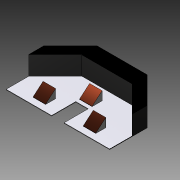
# Autodesk Inventor part: Charging Dock
Saved by Autodesk Inventor 2018 (Build 220112000, 112)
## iProperties
Created: 2017-03-09
Part Number: Charging Dock
Material: ABS Plastic
Document SubType Name: Modeling
Designer: Eightfold_Infotech
Density: 1.06 g/cm^3
Appearance: Smooth - White
Author: Eightfold_Infotech
Autodesk Inventor part; units mm, degrees
ref_plane "YZ Plane" through (0, 0, 0) normal (1, 0, 0) x (0, 1, 0)
ref_plane "XZ Plane" through (0, 0, 0) normal (0, 1, 0) x (-1, 0, 0)
ref_plane "XY Plane" through (0, 0, 0) normal (0, 0, 1) x (1, 0, 0)
sketch "Sketch1" plane through (0, 0, 0) normal (0, 1, 0) x (-1, 0, 0)
  line L0 (-50, -60.443) -> (50, -60.443)
  line L1 (50, -60.443) -> (50, 19.557)
  line L2 (50, 19.557) -> (-50, 19.557)
  line L3 (-50, 19.557) -> (-50, -60.443)
  line L4 (-50, -60.443) -> (50, 19.557) construction
  line L5 (50, -60.443) -> (-50, 19.557) construction
  line L6 (-250, 190) -> (-150, 190)
  line L7 (-150, 190) -> (-150, 110)
  line L8 (-150, 110) -> (-250, 110)
  line L9 (-250, 110) -> (-250, 190)
  line L10 (-250, 190) -> (-150, 110) construction
  line L11 (-150, 190) -> (-250, 110) construction
  line L12 (0, 214.4175) -> (0, -235.835)
  line L13 (250, 190) -> (150, 190)
  line L14 (150, 190) -> (150, 110)
  line L15 (150, 110) -> (250, 110)
  line L16 (250, 110) -> (250, 190)
  line L17 (250, 190) -> (150, 110) construction
  line L18 (150, 190) -> (250, 110) construction
  point P0 (0, 0)
  point P1 (0, -20.443)
  point P2 (-200, 150)
  point P3 (200, 150)
  dimension "d0" = 100
  dimension "d1" = 80
  dimension "d2" = 20.443
  dimension "d3" = 100
  dimension "d4" = 80
  dimension "d5" = 200
  dimension "d6" = 150
  constraints: 38 end point, 6 midpoint, 5 symmetric about line, 4 parallel, 2 horizontal, 2 perpendicular, 1 vertical
  measures "d0" distance of L2.end L1.end
  measures "d1" distance of L1.end L0.end
  measures "d2" distance of point (0, 0) point (0, -20.443)
  measures "d3" distance of L7.end L8.end
  measures "d4" distance of L6.end L7.end
  measures "d5" horizontal distance of point (0, 0) point (-200, 150)
  measures "d6" vertical distance of point (0, 0) point (-200, 150)
sketch "Sketch2" plane through (0, 0, 0) normal (0, 1, 0) x (-1, 0, 0)
  line L0 (-200, -150) -> (200, -150)
  line L1 (200, -150) -> (200, -200)
  line L2 (-200, -200) -> (-200, -150)
  line L3 (0, -269.3547) -> (0, -73.2831)
  line L4 (200, -200) -> (200, -270)
  line L5 (200, -270) -> (-200, -270)
  line L6 (-200, -270) -> (-200, -200)
  line L7 (200, -150) -> (412.132, 62.132)
  line L8 (200, -150) -> (500, -150) construction
  line L9 (412.132, 62.132) -> (412.132, -57.868)
  line L10 (412.132, -57.868) -> (200, -270)
  line L11 (-200, -150) -> (-412.132, 62.132)
  line L12 (-412.132, 62.132) -> (-412.132, -57.868)
  line L13 (-412.132, -57.868) -> (-200, -270)
  point P0 (0, 0)
  point P1 (0, -175)
  point P2 (412.5, 61.0149)
  dimension "d9" = 400
  dimension "d10" = 50
  dimension "d39" = 70
  dimension "d40" = 200
  dimension "d41" = 45
  dimension "d42" = 120
  dimension "d43" = 150
  dimension "d51" = 300
  constraints: 28 end point, 3 perpendicular, 3 vertical, 2 horizontal, 2 symmetric about line, 1 equal length, 1 parallel
  measures "d9" distance of L1.end L2.start
  measures "d10" distance of L0.end L1.end
  measures "d39" distance of L1.end L4.end
  measures "d40" distance from line of L1 point (0, 0)
  measures "d41" angle of L8 L7
  measures "d42" distance of L7.end L9.end
  measures "d43" distance from line of point (0, 0) L0
  measures "d51" distance of L9.end L4.end
extrude "Extrusion2" add sketch "Sketch2" along normal blind 150
fillet "Fillet1" radius 3 1 edges at (0, 150, -150)
extrude "Extrusion6" add sketch "Sketch1" along normal blind 70
sketch "Sketch6" plane through (250, 2, 110) normal (1, 0, 0) x (0, 0, -1)
  line L0 (0, -2) -> (0, 68) projected
  line L1 (-80, 68) -> (0, 68) projected
  line L2 (-80, -2) -> (-80, 68) projected
  line L3 (0, -2) -> (0, 68) projected
  line L4 (-80, -2) -> (-80, 68) projected
  line L5 (-80, 68) -> (0, 68)
  line L6 (-80, 33) -> (-80, 68)
  line L7 (0, 68) -> (-80, 0)
  line L8 (-80, 33) -> (-80, 0)
  line L9 (0, -2) -> (-80, -2) projected
  point P0 (110, -2)
  point P1 (0, 0)
  constraints: 8 end point, 2 collinear, 1 midpoint, 1 perpendicular
extrude "Extrusion7" cut sketch "Sketch6" against normal through all contours L7 L2 L1
sketch "Sketch7" plane through (50, 2, -60.443) normal (1, 0, 0) x (0, 0, -1)
  line L0 (0, -2) -> (0, 68) projected
  line L1 (-80, 68) -> (0, 68) projected
  line L2 (-80, -2) -> (-80, 68) projected
  line L3 (-80, 33) -> (-80, 68)
  line L4 (-80, 68) -> (0, 68) projected
  line L5 (-80, 68) -> (0, 68)
  line L6 (0, 68) -> (-80, 0)
  line L7 (-80, 0) -> (-80, 33)
  line L8 (-80, -2) -> (0, -2) projected
  point P0 (-60.443, -2)
  constraints: 8 end point, 2 collinear, 1 horizontal, 1 midpoint
extrude "Extrusion8" cut sketch "Sketch7" against normal up to surface (100 mm away) contours L6 L2 L1
sketch "Sketch8" plane through (0, 0, 0) normal (0, -1, 0) x (1, 0, 0)
  line L0 (50, 19.557) -> (50, -60.443) projected
  line L1 (50, -60.443) -> (-50, -60.443) projected
  line L2 (-50, -60.443) -> (-50, 19.557) projected
  line L3 (-50, 19.557) -> (50, 19.557) projected
  line L4 (-150, 190) -> (-150, 110) projected
  line L5 (-150, 110) -> (-250, 110) projected
  line L6 (-250, 110) -> (-250, 190) projected
  line L7 (-250, 190) -> (-150, 190) projected
  line L8 (150, 190) -> (250, 190) projected
  line L9 (250, 190) -> (250, 110) projected
  line L10 (250, 110) -> (150, 110) projected
  line L11 (150, 110) -> (150, 190) projected
  line L12 (412.132, -57.868) -> (200, -270) projected
  line L13 (200, -270) -> (-200, -270) projected
  line L14 (-200, -270) -> (-412.132, -57.868) projected
  line L15 (-412.132, -57.868) -> (-412.132, 62.132) projected
  line L16 (-412.132, 62.132) -> (-200, -150) projected
  line L17 (-200, -150) -> (200, -150) projected
  line L18 (200, -150) -> (412.132, 62.132) projected
  line L19 (412.132, 62.132) -> (412.132, -57.868) projected
  line L20 (-412.132, 62.132) -> (-412.132, 242.132)
  line L21 (412.132, 62.132) -> (412.132, 242.132)
  line L22 (-412.132, 62.132) -> (-412.132, -57.868)
  line L23 (-412.132, -57.868) -> (-200, -270)
  line L24 (-200, -270) -> (200, -270)
  line L25 (200, -270) -> (412.132, -57.868)
  line L26 (412.132, -57.868) -> (412.132, 62.132)
  line L27 (50, 242.132) -> (50, 49.557)
  line L28 (50, 49.557) -> (-50, 49.557)
  line L29 (-50, 49.557) -> (-50, 242.132)
  line L30 (412.132, 242.132) -> (50, 242.132)
  line L31 (-50, 242.132) -> (-412.132, 242.132)
  dimension "d45" = 180
  dimension "d46" = 180
  dimension "d47" = 100
  dimension "d48" = 30
  constraints: 24 end point, 5 equal length, 1 point on line, 1 vertical
  measures "d45" distance of L15.end L20.end
  measures "d46" distance of L18.end L21.end
  measures "d47" distance of L27.end L28.end
  measures "d48" distance between parallel lines of L28 L3
extrude "Extrusion9" add sketch "Sketch8" along normal blind 4 contours L0 L1 L2 L3 | L4 L5 L6 L7 | L8 L9 L10 L11 | L12 L13 L14 L15 L16 L17 L18 L19 | L18 L17 L16 L20 L31 L29 L28 L27 L30 L21
sketch "Sketch9" plane through (0, -4, 0) normal (0, -1, 0) x (1, 0, 0)
  line L0 (200, -270) -> (-200, -270) projected
  line L1 (-200, -270) -> (-412.132, -57.868) projected
  line L2 (-412.132, -57.868) -> (-412.132, 242.132) projected
  line L3 (-412.132, 242.132) -> (-50, 242.132) projected
  line L4 (-50, 242.132) -> (-50, 49.557) projected
  line L5 (-50, 49.557) -> (50, 49.557) projected
  line L6 (50, 49.557) -> (50, 242.132) projected
  line L7 (50, 242.132) -> (412.132, 242.132) projected
  line L8 (412.132, 242.132) -> (412.132, -57.868) projected
  line L9 (412.132, -57.868) -> (200, -270) projected
  line L10 (200, -270) -> (-200, -270) projected
  line L11 (-200, -270) -> (-412.132, -57.868) projected
  line L12 (-412.132, -57.868) -> (-412.132, 242.132) projected
  line L13 (-412.132, 242.132) -> (-50, 242.132) projected
  line L14 (-50, 242.132) -> (-50, 49.557) projected
  line L15 (-50, 49.557) -> (50, 49.557) projected
  line L16 (50, 49.557) -> (50, 242.132) projected
  line L17 (50, 242.132) -> (412.132, 242.132) projected
  line L18 (412.132, 242.132) -> (412.132, -57.868) projected
  line L19 (412.132, -57.868) -> (200, -270) projected
  line L20 (200, -270) -> (-200, -270) projected
  line L21 (-200, -270) -> (-412.132, -57.868) projected
  line L22 (-412.132, -57.868) -> (-412.132, 242.132) projected
  line L23 (-412.132, 242.132) -> (-50, 242.132) projected
  line L24 (-50, 242.132) -> (-50, 49.557) projected
  line L25 (-50, 49.557) -> (50, 49.557) projected
  line L26 (50, 49.557) -> (50, 242.132) projected
  line L27 (50, 242.132) -> (412.132, 242.132) projected
  line L28 (412.132, 242.132) -> (412.132, -57.868) projected
  line L29 (412.132, -57.868) -> (200, -270) projected
  line L30 (250, 110) -> (250, 190) projected
  line L31 (50, 19.557) -> (50, -60.443) projected
  line L32 (-50, 19.557) -> (50, 19.557) projected
  line L33 (-50, -60.443) -> (-50, 19.557) projected
  line L34 (50, -60.443) -> (-50, -60.443) projected
  line L35 (-150, 110) -> (-150, 190) projected
  line L36 (-150, 190) -> (-250, 190) projected
  line L37 (-250, 190) -> (-250, 110) projected
  line L38 (-250, 110) -> (-150, 110) projected
  line L39 (250, 190) -> (150, 190) projected
  line L40 (150, 190) -> (150, 110) projected
  line L41 (150, 110) -> (250, 110) projected
  line L42 (250, 110) -> (250, 190) projected
  line L43 (200, -150) -> (412.132, 62.132) projected
  line L44 (-200, -150) -> (200, -150) projected
  line L45 (-412.132, 62.132) -> (-200, -150) projected
  line L46 (-412.132, 242.132) -> (-412.132, 62.132) projected
  line L47 (-50, 242.132) -> (-412.132, 242.132) projected
  line L48 (-50, 49.557) -> (-50, 242.132) projected
  line L49 (50, 49.557) -> (-50, 49.557) projected
  line L50 (50, 242.132) -> (50, 49.557) projected
  line L51 (412.132, 242.132) -> (50, 242.132) projected
  line L52 (412.132, 62.132) -> (412.132, 242.132) projected
  line L53 (50, 19.557) -> (50, -60.443) projected
  line L54 (-50, 19.557) -> (50, 19.557) projected
  line L55 (-50, -60.443) -> (-50, 19.557) projected
  line L56 (50, -60.443) -> (-50, -60.443) projected
  line L57 (-150, 110) -> (-150, 190) projected
  line L58 (-150, 190) -> (-250, 190) projected
  line L59 (-250, 190) -> (-250, 110) projected
  line L60 (-250, 110) -> (-150, 110) projected
  line L61 (250, 190) -> (150, 190) projected
  line L62 (150, 190) -> (150, 110) projected
  line L63 (150, 110) -> (250, 110) projected
  line L64 (250, 110) -> (250, 190) projected
  line L65 (200, -150) -> (412.132, 62.132) projected
  line L66 (-200, -150) -> (200, -150) projected
  line L67 (-412.132, 62.132) -> (-200, -150) projected
  line L68 (-412.132, 242.132) -> (-412.132, 62.132) projected
  line L69 (-50, 242.132) -> (-412.132, 242.132) projected
  line L70 (-50, 49.557) -> (-50, 242.132) projected
  line L71 (50, 49.557) -> (-50, 49.557) projected
  line L72 (50, 242.132) -> (50, 49.557) projected
  line L73 (412.132, 242.132) -> (50, 242.132) projected
  line L74 (412.132, 62.132) -> (412.132, 242.132) projected
  circle A0 centre (242.5, 150) radius 2
  circle A1 centre (242.5, 130) radius 2
  line L75 (200, 190) -> (200, 110) construction
  circle A2 centre (157.5, 150) radius 2
  circle A3 centre (157.5, 130) radius 2
  circle A4 centre (42.5, -20.443) radius 2
  circle A5 centre (42.5, -40.443) radius 2
  circle A6 centre (-42.5, -20.443) radius 2
  circle A7 centre (-42.5, -40.443) radius 2
  circle A8 centre (-157.5, 150) radius 2
  circle A9 centre (-157.5, 130) radius 2
  circle A10 centre (-242.5, 150) radius 2
  circle A11 centre (-242.5, 130) radius 2
  point P0 (0, 0)
  point P1 (0, 19.557)
  point P2 (-200, 190)
  dimension "d52" = 4
  dimension "d53" = 40
  dimension "d54" = 7.5
  dimension "d55" = 4
  dimension "d56" = 0
  dimension "d57" = 20
  dimension "d58" = 4
  dimension "d59" = 4
  dimension "d60" = 0
  dimension "d61" = 20
  dimension "d62" = 4
  dimension "d63" = 4
  dimension "d64" = 0
  dimension "d65" = 20
  constraints: 12 centre point, 4 midpoint, 2 end point, 2 symmetric about line, 2 other
  measures "d52" diameter of A0
  measures "d53" distance from line of A0.centre L39
  measures "d54" distance from line of L30 A0.centre
  measures "d55" diameter of A1
  measures "d56" horizontal distance of A0.centre A1.centre
  measures "d57" distance of A1.centre A0.centre
  measures "d58" diameter of A4
  measures "d59" diameter of A5
  measures "d60" horizontal distance of A4.centre A5.centre
  measures "d61" distance of A5.centre A4.centre
  measures "d62" diameter of A8
  measures "d63" diameter of A9
  measures "d64" horizontal distance of A8.centre A9.centre
  measures "d65" distance of A9.centre A8.centre
extrude "Extrusion10" cut sketch "Sketch9" against normal up to surface (4 mm away) contours A0 | A1 | A2 | A3 | A4 | A5 | A6 | A7 | A8 | A9 | A10 | A11
equation "\"d40\" = 0.5 * d9"
body "Solid1"
